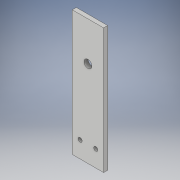
# Autodesk Inventor part: Worm Support
Saved by Autodesk Inventor 2018 (Build 220112000, 112)
## iProperties
Created: 2017-04-14
Part Number: Worm Support
Material: Generic
Document SubType Name: Modeling
Designer: Administrator
Density: 1 g/cm^3
Appearance: Default
Author: Administrator
Autodesk Inventor part; units mm, degrees
ref_plane "YZ Plane" through (0, 0, 0) normal (1, 0, 0) x (0, 1, 0)
ref_plane "XZ Plane" through (0, 0, 0) normal (0, 1, 0) x (-1, 0, 0)
ref_plane "XY Plane" through (0, 0, 0) normal (0, 0, 1) x (1, 0, 0)
sketch "Sketch1" plane through (0, 0, 0) normal (0, 0, 1) x (1, 0, 0)
  line L0 (-25, 0) -> (25, 0)
  line L1 (25, 0) -> (25, 200)
  line L2 (25, 200) -> (-25, 200)
  line L3 (-25, 200) -> (-25, 0)
  circle A0 centre (-12.5, 26.5) radius 3.25
  circle A1 centre (12.5, 26.5) radius 3.25
  point P0 (0, 0)
  dimension "d0" = 50
  dimension "d1" = 200
  dimension "d2" = 6.5
  dimension "d3" = 6.5
  constraints: 8 end point, 2 centre point, 2 parallel, 1 horizontal, 1 perpendicular
  measures "d0" distance of L2.end L1.end
  measures "d1" distance of L1.end L0.end
  measures "d2" diameter of A0
  measures "d3" diameter of A1
extrude "Extrusion1" add sketch "Sketch1" along normal blind 6.5
sketch "Sketch3" plane through (0, 0, 0) normal (0, 0, -1) x (-1, 0, 0)
  circle A0 centre (0, 137.7228) radius 6.35
  point P0 (0, 0)
  dimension "d7" = 12.7
  constraints: 1 centre point
  measures "d7" diameter of A0
hole "Hole1" at (0, 137.7228, 0) direction (0, 0, 1) diameter 12.7 end through all
body "Solid1"
